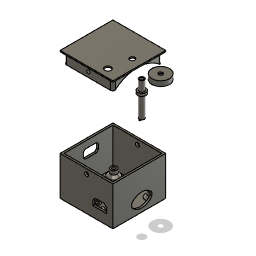
Teensy Audio Case v6 (Autodesk Fusion 360 design; units mm, degrees)
Autodesk Fusion 360 part; units mm, degrees
note: some values were not read from the file. Chosen so that the rebuilt part matches the saved one: a direction.
sketch "Sketch1" plane through (0, 0, 0) normal (0, 1, 0) x (1, 0, 0)
  line L0 (21, 21) -> (-21, 21)
  line L1 (-21, 21) -> (-21, -21)
  line L2 (-21, -21) -> (21, -21)
  line L3 (21, -21) -> (21, 21)
  line L4 (21, 21) -> (-21, -21) construction
  line L5 (-21, 21) -> (21, -21) construction
  line L6 (-19.5, -19.5) -> (19.5, -19.5)
  line L7 (19.5, -19.5) -> (19.5, 19.5)
  line L8 (19.5, 19.5) -> (-19.5, 19.5)
  line L9 (-19.5, 19.5) -> (-19.5, -19.5)
  dimension "d1" = 42
  dimension "d2" = 42
  dimension "d3" = -1.5
  constraint horizontal L0
  constraint perpendicular L0 L1
  constraint parallel L0 L2
  constraint parallel L1 L3
  constraint coincident L4 origin
  constraint coincident L5 origin
  measures "d1" distance of L1.end L2.end
  measures "d2" distance of L0.end L1.end
extrude "Extrude1" add sketch "Sketch1" against normal blind 1 contours L0 L1 L2 L3 | L6 L7 L8 L9 makes body 1
extrude "Extrude2" add sketch "Sketch1" along normal blind 30 bodies 1
sketch "Sketch2" plane through (0, 0, 0) normal (0, 1, 0) x (-1, 0, 0)
  line L0 (19.5, 19.5) -> (-19.5, 19.5)
  line L1 (-19.5, 19.5) -> (-19.5, -19.5)
  line L2 (-19.5, -19.5) -> (19.5, -19.5)
  line L3 (19.5, -19.5) -> (19.5, 19.5)
  line L4 (-17.78, 18.415) -> (17.78, 18.415)
  line L5 (17.78, 18.415) -> (17.78, -18.415)
  line L6 (17.78, -18.415) -> (-17.78, -18.415)
  line L7 (-17.78, -18.415) -> (-17.78, 18.415)
  line L8 (-17.78, 18.415) -> (17.78, -18.415) construction
  line L9 (17.78, 18.415) -> (-17.78, -18.415) construction
  circle A0 centre (14.478, -15.113) radius 2.5
  circle A1 centre (-15.28, -15.113) radius 2.5
  circle A2 centre (-2.78, 15.113) radius 2.5
  dimension "d8" = 35.56
  dimension "d9" = 36.83
  dimension "d10" = 5
  dimension "d11" = 5
  dimension "d12" = 5
  dimension "d13" = 3.302
  dimension "d14" = 3.302
  dimension "d15" = 3.302
  dimension "d16" = 2.5
  dimension "d17" = 15
  dimension "d18" = 3.302
  constraint horizontal L4
  constraint perpendicular L4 L5
  constraint parallel L4 L6
  constraint parallel L5 L7
  constraint coincident L8 origin
  constraint coincident L9 origin
  measures "d8" distance of L5.end L6.end
  measures "d9" distance of L4.end L5.end
  measures "d10" diameter of A0
  measures "d11" diameter of A1
  measures "d12" diameter of A2
  measures "d13" distance of L5 A0.centre
  measures "d14" distance of L6 A0.centre
  measures "d15" distance of L6 A1.centre
  measures "d16" distance of L7 A1.centre
  measures "d17" distance of L7 A2.centre
  measures "d18" distance of L4 A2.centre
extrude "Extrude3" add sketch "Sketch2" along normal blind 5 contours A1 | A0 | A2 bodies 1
sketch "Sketch3" plane through (0, 5, 0) normal (0, 1, 0) x (-1, 0, 0)
  circle A0 centre (14.478, -15.113) radius 2.5
  circle A1 centre (-15.28, -15.113) radius 2.5
  circle A2 centre (-2.78, 15.113) radius 2.5
  circle A3 centre (14.478, -15.113) radius 1.3
  circle A4 centre (-15.28, -15.113) radius 1.3
  circle A5 centre (-2.78, 15.113) radius 1.3
  dimension "d21" = 2.6
  dimension "d22" = 2.6
  dimension "d23" = 2.6
  constraint concentric A0 A3
  constraint concentric A1 A4
  constraint concentric A2 A5
  measures "d21" diameter of A3
  measures "d22" diameter of A4
  measures "d23" diameter of A5
extrude "Extrude4" cut sketch "Sketch3" against normal blind 5 contours A3 | A4 | A5 bodies 1
chamfer "Chamfer1" distance 2 angle 45 3 edges at (-12.1472, 0, -14.209) (17.6108, 0, -14.209) (5.1108, 0, 16.017) on bodies 1
sketch "Sketch4" plane through (-21, 0, 0) normal (-1, 0, 0) x (0, 0, 1)
  line L0 (-21, 30) -> (-21, -1)
  line L1 (-21, -1) -> (21, -1)
  line L2 (21, -1) -> (21, 30)
  line L3 (21, 30) -> (-21, 30)
  circle A0 centre (13.5, 9.5) radius 5
  line L4 (4, 24.5) -> (-8, 24.5)
  line L5 (-8, 24.5) -> (-8, 17.5)
  line L6 (-8, 17.5) -> (4, 17.5)
  line L7 (4, 17.5) -> (4, 24.5)
  line L8 (4, 24.5) -> (-8, 17.5) construction
  line L9 (-8, 24.5) -> (4, 17.5) construction
  line L10 (0, 30) -> (0, -1) construction
  line L11 (13.5, 9.5) -> (13.5, 30) construction
  line L12 (13.5, 16.5) -> (10.0007, 13.0714)
  line L13 (13.5, 16.5) -> (16.9993, 13.0714)
  point P0 (-2, 21)
  dimension "d27" = 10.5
  dimension "d28" = 10
  dimension "d29" = 7.5
  dimension "d30" = 22
  dimension "d31" = 7
  dimension "d32" = 12
  dimension "d36" = 7
  dimension "d51" = 2
  constraint horizontal L4
  constraint perpendicular L4 L5
  constraint parallel L4 L6
  constraint parallel L5 L7
  constraint coincident L8 P0
  constraint coincident L9 P0
  constraint midpoint L3 L10.start
  constraint midpoint L1 L10.end
  constraint coincident A0.centre L11.start
  constraint coincident L3 L11.end
  constraint perpendicular L3 L11
  constraint coincident L11 L12.start
  constraint coincident A0 L12.end
  constraint coincident A0 L13.end
  constraint tangent A0 L12
  constraint tangent A0 L13
  measures "d27" distance of L1 A0.centre
  measures "d28" diameter of A0
  measures "d29" distance of L2 A0.centre
  measures "d30" distance of L1 P0
  measures "d31" distance of L4.start L6.end
  measures "d32" distance of L5.end L6.end
  measures "d36" distance of A0.centre L12.start
  measures "d51" distance of P0 L10
extrude "Extrude5" cut sketch "Sketch4" against normal up to surface (1.5 mm away) contours A0 | A0 L12 L13 | L4 L5 L6 L7 bodies 1
chamfer "Chamfer2" distance 1.5 angle 45 4 edges at (-20.25, 24.5, -8) (-20.25, 24.5, 4) (-20.25, 17.5, -8) (-20.25, 17.5, 4) on bodies 1
sketch "Sketch5" plane through (0, 0, 21) normal (0, 0, 1) x (1, 0, 0)
  line L0 (-21, 30) -> (-21, -1)
  line L1 (-21, -1) -> (21, -1)
  line L2 (21, -1) -> (21, 30)
  line L3 (21, 30) -> (-21, 30)
  line L4 (5, 7) -> (16, 7)
  line L5 (16, 7) -> (16, 13)
  line L6 (16, 13) -> (5, 13)
  line L7 (5, 13) -> (5, 7)
  line L8 (0, 30) -> (0, -1) construction
  circle A0 centre (0, 26.2) radius 1.6
  dimension "d37" = 8
  dimension "d38" = 14
  dimension "d39" = 5
  dimension "d40" = 16
  dimension "d58" = 3.2
  dimension "d59" = 3.8
  constraint horizontal L4
  constraint vertical L5
  constraint horizontal L6
  constraint vertical L7
  constraint midpoint L3 L8.start
  constraint midpoint L1 L8.end
  constraint coincident L8 A0.centre
  measures "d37" distance of L1 L4
  measures "d38" distance of L1 L6
  measures "d39" distance of L2 L5
  measures "d40" distance of L2 L7
  measures "d58" diameter of A0
  measures "d59" distance of L3 A0.centre
extrude "Extrude6" cut sketch "Sketch5" against normal up to surface (1.5 mm away) contours L4 L5 L6 L7 bodies 1
extrude "Extrude10" cut sketch "Sketch5" against normal up to surface (42 mm away) contours A0 bodies 1
chamfer "Chamfer3" distance 2 angle 45 2 edges at (16, 13, 20.25) (5, 13, 20.25) on bodies 1
sketch "Sketch6" plane through (21, 0, 0) normal (1, 0, 0) x (0, 0, -1)
  line L0 (-21, 30) -> (-21, -1)
  line L1 (-21, -1) -> (21, -1)
  line L2 (21, -1) -> (21, 30)
  line L3 (21, 30) -> (-21, 30)
  line L4 (-6, 9) -> (10, 9)
  line L5 (10, 9) -> (10, 6)
  line L6 (10, 6) -> (-6, 6)
  line L7 (-6, 6) -> (-6, 9)
  line L8 (0, -1) -> (0, 30) construction
  arc A0 (10, 9) -> (-6, 9) centre (2, 3) ccw
  arc A1 (-6, 6) -> (10, 6) centre (2, 12) ccw
  point P0 (2, 9)
  dimension "d44" = 7
  dimension "d45" = 10
  dimension "d46" = 16
  dimension "d47" = 6
  dimension "d48" = 6
  dimension "d94" = 2
  constraint horizontal L4
  constraint vertical L5
  constraint horizontal L6
  constraint vertical L7
  constraint midpoint L1 L8.start
  constraint midpoint L3 L8.end
  constraint midpoint L4 P0
  measures "d44" distance of L1 L6
  measures "d45" distance of L1 L4
  measures "d46" distance of L5.end L6.end
  measures "d47" distance of L6 A1.centre
  measures "d48" distance of L4 A0.centre
  measures "d94" distance of L8 P0
extrude "Extrude7" cut sketch "Sketch6" against normal up to surface (1.5 mm away) contours L4 A0 | L4 L5 L6 L7 | L6 A1 bodies 1
ref_plane "WorkPlane1" through (0, 100, 0) normal (0, 1, 0) x (0, 0, 1)
sketch "Sketch7" plane through (0, 100, 0) normal (0, 1, 0) x (1, 0, 0)
  line L0 (-19.5, -19.5) -> (-19.5, 19.5)
  line L1 (-19.5, 19.5) -> (19.5, 19.5)
  line L2 (19.5, 19.5) -> (19.5, -19.5)
  line L3 (19.5, -19.5) -> (-19.5, -19.5)
  line L4 (21, -21) -> (21, 21)
  line L5 (21, 21) -> (-21, 21)
  line L6 (-21, 21) -> (-21, -21)
  line L7 (-21, -21) -> (21, -21)
  line L8 (18, -18) -> (-18, -18)
  line L9 (-18, -18) -> (-18, 18)
  line L10 (-18, 18) -> (18, 18)
  line L11 (18, 18) -> (18, -18)
  dimension "d53" = 1.5
extrude "Extrude8" add sketch "Sketch7" along normal blind 1 separate body contours L0 L1 L2 L3 | L4 L5 L6 L7 | L8 L9 L10 L11 makes body 2
extrude "Extrude9" add sketch "Sketch7" against normal blind 8 contours L0 L1 L2 L3 bodies 2
sketch "Sketch8" plane through (-19.5, 0, 0) normal (-1, 0, 0) x (0, 0, 1)
  line L0 (19.5, 100) -> (-19.5, 100)
  line L1 (-19.5, 100) -> (-19.5, 92)
  line L2 (-19.5, 92) -> (19.5, 92)
  line L3 (19.5, 92) -> (19.5, 100)
  arc A0 (18, 92) -> (-18, 92) centre (0, 71.8754) ccw
  dimension "d62" = 1.5
  dimension "d63" = 1.5
  dimension "d64" = 27
  constraint coincident L2 A0.start
  constraint coincident L2 A0.end
  measures "d62" distance of L1.end A0.end
  measures "d63" distance of L2.end A0.start
  measures "d64" radius of A0
extrude "Extrude11" cut sketch "Sketch8" against normal through all contours L2 A0 bodies 2
chamfer "Chamfer4" distance 6 angle 45 2 edges at (0, 100, -18) (0, 100, 18) on bodies 2
sketch "Sketch9" plane through (0, 0, 19.5) normal (0, 0, 1) x (1, 0, 0)
  line L0 (19.5, 100) -> (-19.5, 100)
  line L1 (-19.5, 100) -> (-19.5, 92)
  line L2 (-19.5, 92) -> (19.5, 92)
  line L3 (19.5, 92) -> (19.5, 100)
  line L4 (0, 100) -> (0, 92) construction
  circle A0 centre (0, 96) radius 1.35
  dimension "d67" = 2.7
  constraint midpoint L0 L4.start
  constraint midpoint L2 L4.end
  constraint midpoint L4 A0.centre
  measures "d67" diameter of A0
extrude "Extrude12" cut sketch "Sketch9" against normal through all contours A0 bodies 2
sketch "Sketch10" plane through (0, 101, 0) normal (0, 1, 0) x (-1, 0, 0)
  line L0 (21, 21) -> (-21, 21)
  line L1 (-21, 21) -> (-21, -21)
  line L2 (-21, -21) -> (21, -21)
  line L3 (21, -21) -> (21, 21)
  circle A0 centre (-13.5, -2) radius 2
  line L4 (-21, -21) -> (21, -21)
  line L5 (21, 0) -> (-21, 0) construction
  circle A1 centre (-10.5, 14.5) radius 2.5
  dimension "d69" = 4
  dimension "d70" = 7.5
  dimension "d72" = 2
  dimension "d73" = 10.5
  dimension "d74" = 6.5
  dimension "d75" = 5
  constraint midpoint L3 L5.start
  constraint midpoint L1 L5.end
  measures "d69" diameter of A0
  measures "d70" distance of L1 A0.centre
  measures "d72" distance of A0.centre L5
  measures "d73" distance of L1 A1.centre
  measures "d74" distance of L0 A1.centre
  measures "d75" diameter of A1
extrude "Extrude13" cut sketch "Sketch10" against normal blind 11 contours A0 | A1 bodies 2
sketch "Sketch11" plane through (0, 92, 0) normal (0, -1, 0) x (1, 0, 0)
  line L0 (-19.5, 18) -> (-18, 18)
  line L1 (-18, 18) -> (18, 18)
  line L2 (18, 18) -> (19.5, 18)
  line L3 (19.5, 18) -> (19.5, 19.5)
  line L4 (19.5, 19.5) -> (-19.5, 19.5)
  line L5 (-19.5, 19.5) -> (-19.5, 18)
  line L6 (5, 18) -> (18, 18)
  line L7 (18, 18) -> (18, 12)
  line L8 (18, 12) -> (5, 12)
  line L9 (5, 12) -> (5, 18)
  line L10 (18, 18) -> (18, 12)
  dimension "d78" = 13
  dimension "d79" = 6
  constraint horizontal L6
  constraint vertical L7
  constraint horizontal L8
  constraint vertical L9
  constraint coincident L1 L6.start
  constraint collinear L7 L10
  measures "d78" distance of L7 L9
  measures "d79" distance of L6 L8
extrude "Extrude14" cut sketch "Sketch11" against normal up to surface (8 mm away) contours L1 L6 L7 L8 L9 L10 bodies 2
sketch "Sketch12" plane through (0, 100, 0) normal (0, 1, 0) x (1, 0, 0)
  circle A0 centre (38, -15) radius 3.25
  circle A1 centre (38, -15) radius 2
  dimension "d82" = 6.5
  dimension "d83" = 4
  constraint concentric A0 A1
  measures "d82" diameter of A0
  measures "d83" diameter of A1
extrude "Extrude15" add sketch "Sketch12" along normal blind 8 separate body contours A1 makes body 3
extrude "Extrude16" add sketch "Sketch12" against normal blind 2 contours A0 | A1 bodies 3
extrude "Extrude17" add sketch "Sketch12" against normal blind 19 contours A1 bodies 3
sketch "Sketch13" plane through (0, 81, 0) normal (0, -1, 0) x (1, 0, 0)
  circle A0 centre (38, 15) radius 2
  line L0 (37.7, 16.9774) -> (37.7, 13.0226)
  line L1 (38.3, 13.0226) -> (38.3, 16.9774)
  line L2 (38.3, 16.9774) -> (37.7, 13.0226) construction
  line L3 (38.3, 13.0226) -> (37.7, 16.9774) construction
  point P0 (38, 15)
  point P1 (38, 15)
  dimension "d90" = 0.6
  constraint coincident A0 L0.start
  constraint coincident A0 L0.end
  constraint vertical L0
  constraint coincident A0 L1.start
  constraint coincident A0 L1.end
  constraint parallel L0 L1
  constraint midpoint L3 P1
  constraint coincident P1 P0
  measures "d90" distance of L0 L1
extrude "Extrude18" add sketch "Sketch13" along normal blind 1 contours A0 L0 L1 bodies 3
fillet "Fillet1" radius 2 4 edges at (-19.5, 96, 19.5) (19.5, 96, 19.5) (19.5, 96, -19.5) (-19.5, 96, -19.5) on bodies 2
sketch "Sketch14" plane through (0, 108, 0) normal (0, 1, 0) x (-1, 0, 0)
  circle A0 centre (-38, 15) radius 2
  circle A1 centre (-38, 15) radius 1.35
  dimension "d97" = 2.7
  constraint concentric A0 A1
  measures "d97" diameter of A1
extrude "Extrude19" cut sketch "Sketch14" against normal blind 6 contours A1 bodies 3
sketch "Sketch15" plane through (0, 100, 0) normal (0, 1, 0) x (1, 0, 0)
  circle A0 centre (38, 0) radius 7
  dimension "d101" = 14
  measures "d101" diameter of A0
extrude "Extrude20" add sketch "Sketch15" along normal blind 4 separate body makes body 4
sketch "Sketch16" plane through (0, 100, 0) normal (0, -1, 0) x (1, 0, 0)
  circle A0 centre (38, 0) radius 7
  circle A1 centre (38, 0) radius 2.25
  circle A2 centre (38, 0) radius 1.6
  dimension "d104" = 4.5
  dimension "d105" = 3.2
  constraint concentric A0 A1
  constraint concentric A1 A2
  measures "d104" diameter of A1
  measures "d105" diameter of A2
extrude "Extrude21" cut sketch "Sketch16" against normal through all contours A2 bodies 4
extrude "Extrude22" cut sketch "Sketch16" against normal blind 3 contours A1 bodies 4
named bodies: "Teensy Audio Case Bottom", "Teensy Audio Case Top", "Teensy Audio Case Volume Rod", "Teensy Audio Case Volume Knob"
